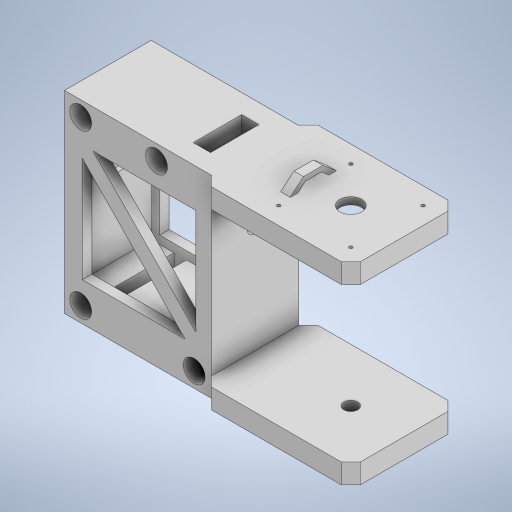
# Autodesk Inventor part: Arm_4_Wholed
Saved by Autodesk Inventor 2023 (Build 270158000, 158)
## iProperties
Created: 2025-02-16
Part Number: Arm_4_Wholed
Material: Generic
Document SubType Name: Modeling
Designer: Swoby
Density: 1 g/cm^3
Appearance: Default
Author: Swoby
Autodesk Inventor part; units mm, degrees
ref_plane "YZ Plane" through (0, 0, 0) normal (1, 0, 0) x (0, 1, 0)
ref_plane "XZ Plane" through (0, 0, 0) normal (0, 1, 0) x (-1, 0, 0)
ref_plane "XY Plane" through (0, 0, 0) normal (0, 0, 1) x (1, 0, 0)
sketch "Sketch1" plane through (0, 0, 0) normal (0, 0, 1) x (1, 0, 0)
  line L0 (40.6, 10.65) -> (40.6, -30.95)
  line L1 (0, -30.95) -> (0, 10.65)
  line L2 (0, 0) -> (-3.1, 0)
  line L3 (-3.1, 0) -> (-3.1, 5)
  line L4 (-3.1, 5) -> (-1.6, 5)
  line L5 (-1.6, 5) -> (-1.6, 7.4)
  line L6 (-1.6, 7.4) -> (0, 7.4)
  line L7 (0, 7.4) -> (0, 0)
  line L8 (7.1, 10.65) -> (7.1, 18.15)
  line L9 (7.1, 18.15) -> (11, 18.15)
  line L10 (11, 18.15) -> (11, 10.65)
  line L11 (31.3, 10.65) -> (31.3, 20.15)
  line L12 (31.3, 20.15) -> (36.7, 20.15)
  line L13 (36.7, 20.15) -> (36.7, 10.65)
  line L14 (7.1, -30.95) -> (7.1, -38.45)
  line L15 (7.1, -38.45) -> (11, -38.45)
  line L16 (11, -38.45) -> (11, -30.95)
  line L17 (0, 10.65) -> (7.1, 10.65)
  line L18 (40.6, -30.95) -> (11, -30.95)
  line L19 (7.1, -30.95) -> (0, -30.95)
  line L20 (11, 10.65) -> (31.3, 10.65)
  line L21 (36.7, 10.65) -> (40.6, 10.65)
  line L22 (31.3, 20.15) -> (-3.1, 20.15)
  line L23 (-3.1, 20.15) -> (-3.1, 5)
  line L24 (-3.1, 0) -> (-3.1, -40.45)
  line L25 (43.1, -40.45) -> (43.1, 20.15)
  line L26 (43.1, 20.15) -> (36.7, 20.15)
  line L27 (40.6, 0) -> (43.1, 0)
  line L28 (43.1, 0) -> (43.1, 2.5)
  line L29 (43.1, 2.5) -> (40.6, 2.5)
  line L30 (40.6, 2.5) -> (40.6, 0)
  line L31 (-3.1, -40.45) -> (43.1, -40.45)
  line L32 (31.3, 10.65) -> (36.7, 10.65)
  point P0 (-3.1, -38.45)
  dimension "d0" = 41.6
  dimension "d1" = 40.6
  dimension "d2" = 1.6
  dimension "d3" = 1.5
  dimension "d4" = 10
  dimension "d5" = 14.8
  dimension "d6" = 7.5
  dimension "d7" = 7.5
  dimension "d8" = 7.1
  dimension "d9" = 3.9
  dimension "d10" = 40.6
  dimension "d11" = 10.65
  dimension "d12" = 3.9
  dimension "d13" = 5.4
  dimension "d14" = 2
  dimension "d15" = 2.5
  dimension "d16" = 2.5
  dimension "d17" = 2
  constraints: 66 end point, 19 perpendicular, 13 point on line, 9 parallel, 7 horizontal, 3 collinear, 3 vertical, 1 coincident
  measures "d0" distance of L1.start L1.end
  measures "d1" distance of L1.end L0.start
  measures "d2" distance of L6.start L7.start
  measures "d3" distance of L3.end L5.start
  measures "d4" diameter of L4 L2
  measures "d5" diameter of L6 L2
  measures "d6" distance of L8.start L8.end
  measures "d7" distance of L14.start L15.start
  measures "d8" distance from line of L8 L1.end
  measures "d9" distance of L8.end L10.start
  measures "d10" distance between parallel lines of L0 L1
  measures "d11" distance from line of point (0, 0) L17
  measures "d12" distance of L13.end L0.start
  measures "d13" distance between parallel lines of L13 L11
  measures "d14" distance between parallel lines of L9 L12
  measures "d15" distance between parallel lines of L25 L0
  measures "d16" distance of L29.start L28.start
  measures "d17" distance between parallel lines of L31 L15
extrude "Extrusion1" add sketch "Sketch1" along normal mid plane 21.2 contours L21 L13 L26 L25 L29 L0 | L29 L25 L27 L0 | L27 L25 L31 L24 L2 L1 L19 L14 L15 L16 L18 L0 | L20 L10 L9 L8 L17 L1 L6 L5 L4 L23 L22 L11 | L4 L5 L6 L1 L2 L3
revolve "Revolution1" cut sketch "Sketch1" angle 360 about axis through (0, 0, 0) along (-1, 0, 0) contours L29 L25 L27 L0 | L4 L5 L6 L1 L2 L3
extrude "Extrusion2" add sketch "Sketch1" against normal blind 3 from surface at 10.6 contours L32 L11 L12 L13
sketch "Sketch2" plane through (0, 0, 10.6) normal (0, 0, 1) x (1, 0, 0)
  line L0 (40.6, 10.65) -> (40.6, -30.95) projected
  line L1 (40.6, -30.95) -> (11, -30.95) projected
  line L2 (11, -30.95) -> (11, -38.45) projected
  line L3 (11, -38.45) -> (7.1, -38.45) projected
  line L4 (7.1, -38.45) -> (7.1, -30.95) projected
  line L5 (7.1, -30.95) -> (0, -30.95) projected
  line L6 (0, -30.95) -> (0, 10.65) projected
  line L7 (0, 10.65) -> (7.1, 10.65) projected
  line L8 (7.1, 10.65) -> (7.1, 18.15) projected
  line L9 (7.1, 18.15) -> (11, 18.15) projected
  line L10 (11, 18.15) -> (11, 10.65) projected
  line L11 (11, 10.65) -> (40.6, 10.65) projected
  line L12 (43.1, -40.45) -> (43.1, 20.15) projected
  line L13 (43.1, 20.15) -> (-3.1, 20.15) projected
  line L14 (-3.1, 20.15) -> (-3.1, -40.45) projected
  line L15 (-3.1, -40.45) -> (43.1, -40.45) projected
  point P0 (0, 0)
extrude "Extrusion3" add sketch "Sketch2" along normal blind 3 contours L0 L1 L2 L3 L4 L5 L6 L7 L8 L9 L10 L11 | L15 L14 L13 L12
mirror "Mirror1" about plane through (0, 0, 0) normal (0, 0, 1) of "Extrusion3", "Extrusion2"
sketch "Sketch3" plane through (0, 0, 0) normal (0, 0, 1) x (1, 0, 0)
  circle A0 centre (25.8, 15.4) radius 3.4
  circle A1 centre (2, 15.4) radius 3.4
  circle A2 centre (2, -35.7) radius 3.4
  circle A3 centre (37.6, -35.7) radius 3.4
  circle A4 centre (2, 15.4) radius 2.15
  circle A5 centre (25.8, 15.4) radius 2.15
  circle A6 centre (2, -35.7) radius 2.15
  circle A7 centre (37.6, -35.7) radius 2.15
  circle A8 centre (37.6, -35.7) radius 1.75
  circle A9 centre (2, -35.7) radius 1.75
  circle A10 centre (2, 15.4) radius 1.75
  circle A11 centre (25.8, 15.4) radius 1.75
  line L0 (43.1, 20.15) -> (-3.1, 20.15) projected
  line L1 (43.1, -40.45) -> (43.1, 20.15) projected
  line L2 (-3.1, -40.45) -> (43.1, -40.45) projected
  line L3 (-3.1, 20.15) -> (-3.1, -40.45) projected
  line L4 (11, 10.65) -> (11, 18.15) projected
  line L5 (7.1, 18.15) -> (7.1, 10.65) projected
  line L6 (7.1, 10.65) -> (0, 10.65) projected
  line L7 (11, 18.15) -> (7.1, 18.15) projected
  line L8 (40.6, 10.65) -> (11, 10.65) projected
  line L9 (11, -30.95) -> (40.6, -30.95) projected
  line L10 (0, -30.95) -> (7.1, -30.95) projected
  line L11 (7.1, -30.95) -> (7.1, -38.45) projected
  line L12 (7.1, -38.45) -> (11, -38.45) projected
  line L13 (11, -38.45) -> (11, -30.95) projected
  line L14 (40.6, 10.65) -> (11, 10.65) projected
  line L15 (11, 10.65) -> (11, 18.15) projected
  line L16 (11, 18.15) -> (7.1, 18.15) projected
  line L17 (7.1, 18.15) -> (7.1, 10.65) projected
  line L18 (7.1, 10.65) -> (0, 10.65) projected
  line L19 (0, 10.65) -> (0, -30.95) projected
  line L20 (0, -30.95) -> (7.1, -30.95) projected
  line L21 (7.1, -30.95) -> (7.1, -38.45) projected
  line L22 (7.1, -38.45) -> (11, -38.45) projected
  line L23 (11, -38.45) -> (11, -30.95) projected
  line L24 (11, -30.95) -> (40.6, -30.95) projected
  line L25 (40.6, -30.95) -> (40.6, 10.65) projected
  line L26 (31.3, 20.15) -> (36.7, 20.15) projected
  line L27 (31.3, 10.65) -> (31.3, 20.15) projected
  line L28 (36.7, 10.65) -> (31.3, 10.65) projected
  line L29 (36.7, 20.15) -> (36.7, 10.65) projected
  line L30 (40.6, -2.5) -> (40.6, 2.5) projected
  line L31 (43.1, 2.5) -> (43.1, -2.5) projected
  line L32 (-3.1, -5) -> (-3.1, 5) projected
  line L33 (-1.6, -5) -> (-1.6, 5) projected
  line L34 (-1.6, -7.4) -> (-1.6, 7.4) projected
  line L35 (0, 7.4) -> (0, -7.4) projected
  point P0 (0, 0)
  point P1 (0, 0)
  dimension "d25" = 6.8
  dimension "d28" = 6.8
  dimension "d33" = 6.8
  dimension "d34" = 6.8
  dimension "d40" = 4.3
  dimension "d41" = 4.3
  dimension "d42" = 4.3
  dimension "d43" = 4.3
  dimension "d44" = 3.5
  dimension "d45" = 3.5
  dimension "d46" = 3.5
  dimension "d47" = 3.5
  dimension "d48" = 9.5
  dimension "d49" = 4.75
  dimension "d50" = 4.75
  dimension "d51" = 10.2
  dimension "d52" = 5.1
  dimension "d53" = 5.5
  dimension "d54" = 9.5
  dimension "d55" = 4.75
  dimension "d56" = 4.75
  dimension "d57" = 5.1
  dimension "d58" = 5.5
  constraints: 12 centre point, 8 coincident
  measures "d25" diameter of A0
  measures "d28" diameter of A1
  measures "d33" diameter of A2
  measures "d34" diameter of A3
  measures "d40" diameter of A4
  measures "d41" diameter of A5
  measures "d42" diameter of A6
  measures "d43" diameter of A7
  measures "d44" diameter of A8
  measures "d45" diameter of A9
  measures "d46" diameter of A10
  measures "d47" diameter of A11
  measures "d48" distance between parallel lines of L6 L0
  measures "d49" distance from line of L6 A10.centre
  measures "d50" distance from line of L8 A0.centre
  measures "d51" distance between parallel lines of L5 L3
  measures "d52" distance from line of L5 A10.centre
  measures "d53" distance from line of L27 A0.centre
  measures "d54" distance between parallel lines of L2 L20
  measures "d55" distance from line of L2 A2.centre
  measures "d56" distance from line of L2 A7.centre
  measures "d57" distance from line of L11 A2.centre
  measures "d58" distance from line of L1 A3.centre
extrude "Extrusion4" cut sketch "Sketch3" against normal blind 5 from surface at 13.6 contours A0 | A1 | A2 | A3 | A4 | A5 | A6 | A7 | A8 | A9 | A10 | A11
extrude "Extrusion5" cut sketch "Sketch3" along normal through all contours A8 | A9 | A10 | A11
extrude "Extrusion6" cut sketch "Sketch3" against normal blind 10 contours A4 | A5 | A6 | A7 | A8 | A9 | A10 | A11
sketch "Sketch4" plane through (0, 0, 0) normal (0, 0, 1) x (1, 0, 0)
  line L0 (40.6, 10.65) -> (11, 10.65) projected
  line L1 (11, 10.65) -> (11, 18.15) projected
  line L2 (11, 18.15) -> (7.1, 18.15) projected
  line L3 (7.1, 18.15) -> (7.1, 10.65) projected
  line L4 (7.1, 10.65) -> (0, 10.65) projected
  line L5 (0, 10.65) -> (0, -30.95) construction
  line L6 (0, -30.95) -> (7.1, -30.95) construction
  line L7 (7.1, -30.95) -> (7.1, -38.45) projected
  line L8 (7.1, -38.45) -> (11, -38.45) projected
  line L9 (11, -38.45) -> (11, -30.95) projected
  line L10 (11, -30.95) -> (40.6, -30.95) projected
  line L11 (40.6, -30.95) -> (40.6, 10.65) construction
  line L12 (0, 10.65) -> (40.6, -30.95) construction
  line L13 (0, 10.65) -> (0, -30.95) construction
  line L14 (0, -30.95) -> (40.6, -30.95) construction
  line L15 (34.6668, -28.45) -> (2.5, 4.5091)
  line L16 (2.5, 4.5091) -> (2.5, -28.45)
  line L17 (2.5, -28.45) -> (34.6668, -28.45)
  line L18 (0, 10.65) -> (40.6, 10.65) construction
  line L19 (40.6, -30.95) -> (40.6, 10.65)
  line L20 (0, 10.65) -> (40.6, -30.95) construction
  line L21 (38.1, 8.15) -> (5.9332, 8.15)
  line L22 (5.9332, 8.15) -> (38.1, -24.8091)
  line L23 (38.1, -24.8091) -> (38.1, 8.15)
  point P0 (0, 0)
  dimension "d65" = 2.5
  dimension "d66" = 2.5
  constraints: 24 end point, 2 collinear, 2 perpendicular, 1 vertical, 4 other
  measures "d65" distance between parallel lines of L12 L15
  measures "d66" distance between parallel lines of L18 L21
extrude "Extrusion7" cut sketch "Sketch4" along normal through all both and the other way through all
sketch "Sketch5" plane through (0, 0, 0) normal (0, 1, 0) x (-1, 0, 0)
  circle A0 centre (-73.1, 0) radius 3.4
  line L0 (-73.1, 0) -> (-85.8279, -12.7279) construction
  line L1 (-73.1, 0) -> (-85.8279, 12.7279) construction
  arc A1 (-87.4701, -11.5863) -> (-87.2421, -14.1421) centre (-85.8279, -12.7279) ccw
  arc A2 (-87.2421, 14.1421) -> (-87.4701, 11.5863) centre (-85.8279, 12.7279) ccw
  line L2 (-77.6962, 4.5962) -> (-80.5953, 1.6971) construction
  line L3 (-77.6962, -4.5962) -> (-80.5953, -1.6971) construction
  line L4 (-87.4701, 11.5863) -> (-80.5953, 1.6971)
  line L5 (-80.5953, -1.6971) -> (-87.4701, -11.5863)
  arc A3 (-80.6244, -1.7382) -> (-80.5953, 1.6971) centre (-83.0365, 0) ccw
  line L6 (-85.8279, -12.7279) -> (-87.2421, -14.1421) construction
  line L7 (-85.8279, 12.7279) -> (-87.2421, 14.1421) construction
  circle A4 centre (-84.4137, -11.3137) radius 0.5
  line L8 (-71.4029, -7.4953) -> (-61.5137, -14.3701)
  arc A5 (-61.5137, -14.3701) -> (-58.9579, -14.1421) centre (-60.3721, -12.7279) ccw
  circle A6 centre (-61.7863, -11.3137) radius 0.5
  line L9 (-84.6863, -14.3701) -> (-74.7971, -7.4953)
  arc A7 (-87.2421, -14.1421) -> (-84.6863, -14.3701) centre (-85.8279, -12.7279) ccw
  arc A8 (-71.3618, -7.5244) -> (-74.7971, -7.4953) centre (-73.1, -9.9365) ccw
  line L10 (-65.6047, 1.6971) -> (-58.7299, 11.5863)
  arc A9 (-58.7299, 11.5863) -> (-58.9579, 14.1421) centre (-60.3721, 12.7279) ccw
  circle A10 centre (-61.7863, 11.3137) radius 0.5
  line L11 (-58.7299, -11.5863) -> (-65.6047, -1.6971)
  arc A11 (-58.9579, -14.1421) -> (-58.7299, -11.5863) centre (-60.3721, -12.7279) ccw
  arc A12 (-65.5756, 1.7382) -> (-65.6047, -1.6971) centre (-63.1635, 0) ccw
  line L12 (-74.7971, 7.4953) -> (-84.6863, 14.3701)
  arc A13 (-84.6863, 14.3701) -> (-87.2421, 14.1421) centre (-85.8279, 12.7279) ccw
  circle A14 centre (-84.4137, 11.3137) radius 0.5
  line L13 (-61.5137, 14.3701) -> (-71.4029, 7.4953)
  arc A15 (-58.9579, 14.1421) -> (-61.5137, 14.3701) centre (-60.3721, 12.7279) ccw
  arc A16 (-74.8382, 7.5244) -> (-71.4029, 7.4953) centre (-73.1, 9.9365) ccw
  circle A17 centre (-73.1, 0) radius 2.15
  line L14 (-43.1, -13.6) -> (-43.1, 13.6) projected
  line L15 (-43.1, 0) -> (-73.1, 0) construction
  line L16 (-46.1, -16.7279) -> (-86.8279, -16.7279)
  line L17 (-89.8279, -13.7279) -> (-89.8279, 13.7279)
  line L18 (-86.8279, 16.7279) -> (-46.1, 16.7279)
  line L19 (-43.1, 13.7279) -> (-43.1, -13.7279)
  line L20 (-46.1, -16.7279) -> (-43.1, -13.7279)
  line L21 (-86.8279, -16.7279) -> (-89.8279, -13.7279)
  line L22 (-89.8279, 13.7279) -> (-86.8279, 16.7279)
  line L23 (-46.1, 16.7279) -> (-43.1, 13.7279)
  point P0 (0, 0)
  point P1 (-43.1, -16.7279)
  point P2 (-89.8279, 16.7279)
  point P3 (-89.8279, -16.7279)
  point P4 (-43.1, 16.7279)
  point P5 (-58.9579, -14.1421)
  point P6 (-58.9579, 14.1421)
  point P7 (-87.2421, 14.1421)
  point P8 (-87.2421, -14.1421)
  dimension "d71" = 6.8
  dimension "d74" = 18
  dimension "d75" = 18
  dimension "d76" = 4
  dimension "d77" = 4
  dimension "d78" = 4.1
  dimension "d79" = 6.5
  dimension "d80" = 4.1
  dimension "d81" = 6.5
  dimension "d82" = 1
  dimension "d83" = 2
  dimension "d84" = 360
  dimension "d87" = 4.3
  dimension "d90" = 30
  dimension "d91" = 135
  dimension "d92" = 4
  dimension "d93" = 4
  dimension "d94" = 4
  dimension "d95" = 3
  dimension "d96" = 3
  dimension "d97" = 3
  dimension "d98" = 3
  dimension "d99" = 3
  dimension "d100" = 3
  dimension "d101" = 3
  dimension "d102" = 3
  constraints: 46 end point, 24 point on circle, 18 centre point, 12 point on line, 4 coincident, 4 tangent, 3 perpendicular, 2 collinear, 2 horizontal, 2 parallel, 1 midpoint, 69 other
  measures "d71" diameter of A0
  measures "d74" distance of L0.start L0.end
  measures "d75" distance of L0.start L1.end
  measures "d76" diameter of A1
  measures "d77" diameter of A2
  measures "d78" distance of L2.start L2.end
  measures "d79" distance between parallel lines of L2 L0
  measures "d80" distance of L3.start L3.end
  measures "d81" distance from line of L1 L3.start
  measures "d82" diameter of A4
  measures "d83" distance of L6.start A4.centre
  measures "d87" diameter of A17
  measures "d90" distance of L15.start L15.end
  measures "d91" angle of L15 L0
  measures "d92" distance from line of A5.centre L16
  measures "d93" distance from line of L18 A15.centre
  measures "d94" distance from line of L17 L7.start
  measures "d95" distance of L16.start point (-43.1, -16.728)
  measures "d96" distance of L19.end point (-43.1, -16.728)
  measures "d97" distance of L16.end point (-89.828, -16.728)
  measures "d98" distance of L17.start point (-89.828, -16.728)
  measures "d99" distance of L17.end point (-89.828, 16.728)
  measures "d100" distance of L18.start point (-89.828, 16.728)
  measures "d101" distance of L18.end point (-43.1, 16.728)
  measures "d102" distance of L19.start point (-43.1, 16.728)
ref_plane "Work Plane2" through (-3.1, 13.95, 13.6) normal (0, 1, 0) x (1, 0, 0)
extrude "Extrusion8" add sketch "Sketch5" along normal up to surface (6.2 mm away) from surface at 13.95 contours A0 | L5 A3 L4 A2 A13 L12 A16 L13 A15 A9 L10 A12 L11 A11 A5 L8 A8 L9 A7 A1 | A4 | A6 | A10 | A14 | A17 | L19 L20 L16 L21 L17 L22 L18 L23 L14
ref_plane "Work Plane3" through (-3.1, -10.15, 13.6) normal (0, 1, 0) x (1, 0, 0)
mirror "Mirror2" about plane through (-3.1, -10.15, 13.6) normal (0, 1, 0) of "Extrusion8"
extrude "Extrusion9" cut sketch "Sketch5" along normal through all contours A0 | A4 | A6 | A10 | A14 | A17
extrude "Extrusion10" cut sketch "Sketch5" along normal blind 4 from surface at 13.95 contours L5 A3 L4 A2 A13 L12 A16 L13 A15 A9 L10 A12 L11 A11 A5 L8 A8 L9 A7 A1
extrude "Extrusion11" cut sketch "Sketch5" against normal through all contours A17
ref_plane "Work Plane4" through (59.8279, 13.95, 13.7279) normal (1, 0, 0) x (0, 0, -1)
sketch "Sketch6" plane through (59.8279, 13.95, 13.7279) normal (1, 0, 0) x (0, 0, -1)
  line L0 (27.3279, 6.2) -> (0.1279, 6.2) projected
  line L1 (0, 6.2) -> (0.1279, 6.2) projected
  line L2 (-3, 6.2) -> (0, 6.2) projected
  line L3 (0, 6.2) -> (-3, 6.2) projected
  line L4 (27.4558, 6.2) -> (0, 6.2) projected
  line L5 (30.4558, 6.2) -> (27.4558, 6.2) projected
  line L6 (27.4558, 6.2) -> (30.4558, 6.2) projected
  line L7 (27.3279, 6.2) -> (27.4558, 6.2) projected
  line L8 (21.3279, 6.2) -> (6.1279, 6.2) projected
  line L9 (21.3279, 6.2) -> (6.1279, 6.2) projected
  line L10 (10.3279, 6.2) -> (17.1279, 6.2) projected
  line L11 (24.5416, 6.2) -> (25.5416, 6.2) projected
  line L12 (1.9142, 6.2) -> (2.9142, 6.2) projected
  line L13 (1.9142, 6.2) -> (2.9142, 6.2) projected
  line L14 (24.5416, 6.2) -> (25.5416, 6.2) projected
  line L15 (13.7279, 6.2) -> (13.7279, 8.2) construction
  line L16 (16.2279, 8.2) -> (11.2279, 8.2)
  line L17 (11.2279, 8.2) -> (8.8444, 6.2)
  line L18 (16.2279, 8.2) -> (18.6114, 6.2)
  line L19 (6.5108, 6.2) -> (10.682, 9.7)
  line L20 (10.682, 9.7) -> (16.7739, 9.7)
  line L21 (16.7739, 9.7) -> (20.945, 6.2)
  point P0 (13.7279, -13.95)
  point P1 (18.6114, 6.2)
  point P2 (8.8444, 6.2)
  dimension "d113" = 2
  dimension "d114" = 5
  dimension "d115" = 140
  dimension "d116" = 140
  dimension "d117" = 1.5
  dimension "d118" = 1.5
  dimension "d119" = 1.5
  constraints: 14 end point, 4 point on line, 2 horizontal, 2 midpoint, 2 parallel, 1 vertical
  measures "d113" distance of L15.end L15.start
  measures "d114" distance of L16.start L16.end
  measures "d115" angle of L8 L18
  measures "d116" angle of L8 L17
  measures "d117" distance between parallel lines of L16 L20
  measures "d118" distance between parallel lines of L19 L17
  measures "d119" distance between parallel lines of L21 L18
extrude "Extrusion12" add sketch "Sketch6" along normal mid plane 3 contours L0 L18 L16 L17 L19 L20 L21
equation "\"d7\" = d6"
equation "\"d49\" = 0.5 * d48"
equation "\"d50\" = d49"
equation "\"d52\" = 0.5 * d51"
equation "\"d55\" = 0.5 * d54"
equation "\"d56\" = d55"
equation "\"d57\" = d52"
equation "\"d75\" = d74"
equation "\"d81\" = d79"
equation "\"d93\" = d92"
equation "\"d96\" = d95"
equation "\"d97\" = d95"
equation "\"d98\" = d97"
equation "\"d99\" = d95"
equation "\"d100\" = d99"
equation "\"d101\" = d95"
equation "\"d102\" = d101"
body "Solid1"
